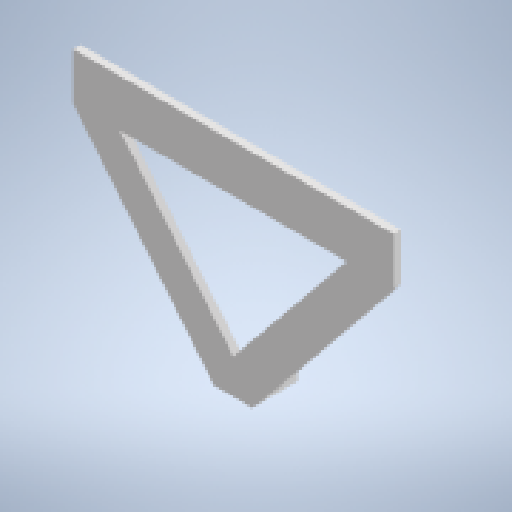
# Autodesk Inventor part: BareCalibrationClipBatteryMount
Saved by Autodesk Inventor 2024 (Build 280153000, 153)
## iProperties
Created: 2024-03-12
Part Number: BareCalibrationClipBatteryMount
Material: Generic
Document SubType Name: Modeling
Designer: jevan
Density: 1 g/cm^3
Appearance: Default
Author: jevan
Autodesk Inventor part; units mm, degrees
ref_plane "YZ Plane" through (0, 0, 0) normal (1, 0, 0) x (0, 1, 0)
ref_plane "XZ Plane" through (0, 0, 0) normal (0, 1, 0) x (-1, 0, 0)
ref_plane "XY Plane" through (0, 0, 0) normal (0, 0, 1) x (1, 0, 0)
sketch "Sketch1" plane through (0, 0, 0) normal (0, 0, 1) x (1, 0, 0)
  line L0 (20.5636, -7.0902) -> (-9.4364, -7.0902)
  line L1 (-9.4364, -7.0902) -> (-9.4364, 33.4098)
  line L2 (-9.4364, 33.4098) -> (20.5636, 33.4098)
  line L3 (20.5636, 33.4098) -> (20.5636, -7.0902)
  line L4 (20.5636, 13.9098) -> (-9.4364, 13.9098)
  line L5 (20.5636, 13.9098) -> (25.5636, 13.9098)
  line L6 (25.5636, 13.9098) -> (25.5636, 18.9098)
  line L7 (25.5636, 18.9098) -> (20.5636, 18.9098)
  line L8 (5.5636, -7.0902) -> (5.5636, 33.4098)
  line L9 (-9.4364, 13.9098) -> (-14.4364, 13.9098)
  line L10 (-14.4364, 13.9098) -> (-14.4364, 18.9098)
  line L11 (-14.4364, 18.9098) -> (-9.4364, 18.9098)
  line L12 (3.0636, -7.0902) -> (3.0636, -9.0902)
  line L13 (3.0636, -9.0902) -> (8.0636, -9.0902)
  line L14 (8.0636, -9.0902) -> (8.0636, -7.0902)
  line L15 (3.0636, -9.0902) -> (-11.9364, 13.9098)
  line L16 (8.0636, -9.0902) -> (23.0636, 13.9098)
  line L17 (-9.4364, 18.9098) -> (20.5636, 18.9098)
  line L18 (17.0943, 13.9098) -> (5.5636, -3.7706)
  line L19 (5.5636, -3.7706) -> (-5.967, 13.9098)
  point P0 (0, 0)
  point P1 (20.5636, 9.5176)
  point P2 (-9.4364, 9.5176)
  point P3 (5.5636, -1.9167)
  point P4 (-9.4364, 13.9098)
  dimension "d0" = 30
  dimension "d1" = 40.5
  dimension "d4" = 5
  dimension "d5" = 5
  dimension "d7" = 2
  dimension "d8" = 5
  dimension "d9" = 2.5
  dimension "d12" = 23
  dimension "d15" = 5
  constraints: 40 end point, 12 point on line, 7 perpendicular, 4 midpoint, 4 symmetric about line, 3 parallel, 2 horizontal, 1 collinear, 1 equal length, 1 vertical
  measures "d0" distance of L0.start L0.end
  measures "d1" distance between parallel lines of L2 L0
  measures "d4" distance between parallel lines of L7 L5
  measures "d5" distance between parallel lines of L3 L6
  measures "d7" distance between parallel lines of L0 L13
  measures "d8" distance between parallel lines of L14 L12
  measures "d9" distance between parallel lines of L8 L12
  measures "d12" distance between parallel lines of L13 L9
  measures "d15" distance between parallel lines of L16 L18
extrude "Extrusion1" add sketch "Sketch1" along normal blind 0.6 contours L14 L13 L12 L0 | L0 L8 L18 L4 L3 L16 | L0 L16 L14 | L0 L15 L1 L4 L19 L8 | L12 L15 L0 | L3 L5 L16 | L8 L17 L3 L4 | L4 L1 L17 L8 | L3 L7 L6 L5 | L15 L9 L1 | L9 L10 L11 L1
extrude "Extrusion2" add sketch "Sketch1" against normal blind 5 contours L14 L13 L12 L0
extrude "Extrusion3" add sketch "Sketch1" against normal blind 6 contours L3 L7 L6 L5 | L9 L10 L11 L1
chamfer "Chamfer1" distance 2.5 distance2 5 2 edges at (-14.4364, 16.4098, 0.6) (25.5636, 16.4098, 0.6) measured on face at (25.0636, 16.4098, 0.6) measured on face at (-13.9364, 16.4098, 0.6)
sketch "Sketch3" plane through (0, 0, -6) normal (0, 0, -1) x (-1, 0, 0)
  line L0 (9.4364, 13.9098) -> (14.4364, 13.9098) projected
  line L1 (9.4364, 13.9098) -> (14.4364, 13.9098)
  line L2 (14.4364, 13.9098) -> (14.4364, 18.9098)
  line L3 (14.4364, 18.9098) -> (9.4364, 18.9098)
  line L4 (9.4364, 18.9098) -> (9.4364, 13.9098)
  line L5 (-20.5636, 13.9098) -> (-23.0636, 13.9098) projected
  line L6 (-25.5636, 18.9098) -> (-25.5636, 13.9098) projected
  line L7 (-20.5636, 13.9098) -> (-25.5636, 13.9098)
  line L8 (-25.5636, 13.9098) -> (-25.5636, 18.9098)
  line L9 (-25.5636, 18.9098) -> (-20.5636, 18.9098)
  line L10 (-20.5636, 18.9098) -> (-20.5636, 13.9098)
  line L11 (-21.5636, 14.9098) -> (-24.5636, 14.9098)
  line L12 (-24.5636, 14.9098) -> (-24.5636, 17.9098)
  line L13 (-24.5636, 17.9098) -> (-21.5636, 17.9098)
  line L14 (-21.5636, 17.9098) -> (-21.5636, 14.9098)
  line L15 (13.4364, 17.9098) -> (13.4364, 14.9098)
  line L16 (13.4364, 14.9098) -> (10.4364, 14.9098)
  line L17 (10.4364, 14.9098) -> (10.4364, 17.9098)
  line L18 (10.4364, 17.9098) -> (13.4364, 17.9098)
  point P0 (0, 0)
  dimension "d23" = 1
  dimension "d24" = 1
  constraints: 32 end point, 8 parallel, 4 perpendicular, 2 horizontal, 6 other
  measures "d23" distance between parallel lines of L10 L14
  measures "d24" distance between parallel lines of L2 L15
extrude "Extrusion4" add sketch "Sketch3" along normal blind 3 contours L11 L12 L13 L14 | L15 L16 L17 L18
chamfer "Chamfer2" distance 0.5 angle 45 8 edges at (23.0636, 17.9098, -9) (24.5636, 16.4098, -9) (21.5636, 16.4098, -9) (23.0636, 14.9098, -9) (-13.4364, 16.4098, -9) (-11.9364, 17.9098, -9) (-10.4364, 16.4098, -9) (-11.9364, 14.9098, -9)
equation "\"d5\" = d4"
equation "\"d9\" = 0.5 * d8"
body "Solid1"
